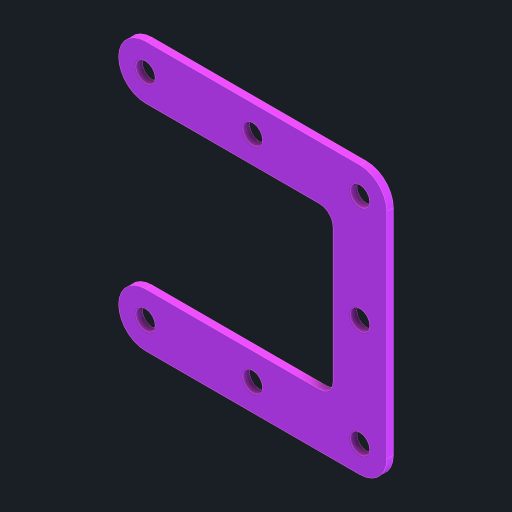
# Autodesk Inventor part: frontgusset
Saved by Autodesk Inventor 2023 (Build 270158000, 158)
## iProperties
Created: 2023-05-11
Part Number: frontgusset
Material: Polycarbonate, Clear
Document SubType Name: Sheet Metal
Designer: reima
Density: 1.2 g/cm^3
Appearance: Magenta
Sheet Metal Rule: Default
Author: reima
Autodesk Inventor part; units mm, degrees
ref_plane "YZ Plane" through (0, 0, 0) normal (1, 0, 0) x (0, 1, 0)
ref_plane "XZ Plane" through (0, 0, 0) normal (0, 1, 0) x (-1, 0, 0)
ref_plane "XY Plane" through (0, 0, 0) normal (0, 0, 1) x (1, 0, 0)
sketch "Sketch1" plane through (0, 0, 0) normal (0, 0, 1) x (1, 0, 0)
  line L0 (-127.5242, -32.3587) -> (-188.9758, -32.3587) projected
  line L1 (-128.9881, -97.1287) -> (-187.5119, -97.1287) projected
  line L2 (-113.8, -97.1287) -> (-113.8, -85.5717) projected
  circle A0 centre (-120.15, -39.9787) radius 2.3114 projected
  circle A1 centre (-120.15, -90.7787) radius 2.3114 projected
  circle A2 centre (-170.95, -90.7787) radius 2.3114 projected
  circle A3 centre (-170.95, -39.9787) radius 2.3114 projected
  circle A4 centre (-158.25, -39.9787) radius 2.3114 projected
  circle A5 centre (-158.25, -90.7787) radius 2.3114 projected
  circle A6 centre (-120.15, -39.9787) radius 6.35
  circle A7 centre (-170.95, -39.9787) radius 6.35
  circle A8 centre (-170.95, -90.7787) radius 6.35
  circle A9 centre (-120.15, -90.7787) radius 6.35
  line L3 (-170.95, -33.6287) -> (-120.15, -33.6287)
  line L4 (-113.8, -39.9787) -> (-113.8, -90.7787)
  line L5 (-120.15, -97.1287) -> (-170.95, -97.1287)
  line L6 (-170.95, -46.3287) -> (-129.675, -46.3287)
  line L7 (-126.5, -49.5037) -> (-126.5, -81.2537)
  line L8 (-129.675, -84.4287) -> (-170.95, -84.4287)
  arc A10 (-126.5, -49.5037) -> (-129.675, -46.3287) centre (-129.675, -49.5037) ccw
  arc A11 (-129.675, -84.4287) -> (-126.5, -81.2537) centre (-129.675, -81.2537) ccw
  circle A12 centre (-170.95, -39.9787) radius 2.3114
  circle A13 centre (-120.15, -39.9787) radius 2.3114
  circle A14 centre (-120.15, -90.7787) radius 2.3114
  circle A15 centre (-170.95, -90.7787) radius 2.3114
  circle A16 centre (-158.25, -90.7787) radius 2.3114
  circle A17 centre (-158.25, -39.9787) radius 2.3114
  point P0 (0, 0)
  dimension "d6" = 12.7
  dimension "d7" = 12.7
  dimension "d8" = 12.7
  dimension "d9" = 12.7
  dimension "d10" = 3.175
  constraints: 12 centre point, 12 end point, 12 point on circle, 10 coincident, 8 tangent, 7 equal radius, 2 point on line, 1 horizontal, 1 perpendicular
  measures "d6" diameter of A6
  measures "d7" diameter of A7
  measures "d8" diameter of A8
  measures "d9" diameter of A9
  measures "d10" radius of A10
extrude "Extrusion1" add sketch "Sketch1" along normal blind 1.5875
sketch "Sketch2" plane through (0, 0, 1.5875) normal (0, 0, 1) x (1, 0, 0)
  circle A0 centre (-158.25, -39.9787) radius 2.3114 projected
  circle A1 centre (-158.25, -39.9787) radius 2.3114
  circle A2 centre (-158.25, -90.7787) radius 2.3114 projected
  circle A3 centre (-158.25, -90.7787) radius 2.3114
  circle A4 centre (-145.55, -90.7787) radius 2.3368
  circle A5 centre (-170.95, -90.7787) radius 2.3114 projected
  circle A6 centre (-145.55, -39.9787) radius 2.3368
  circle A7 centre (-120.15, -65.3787) radius 2.3368
  circle A8 centre (-120.15, -39.9787) radius 2.3114 projected
  line L0 (-113.8, -90.7787) -> (-113.8, -39.9787) projected
  circle A9 centre (-170.95, -39.9787) radius 2.3114 projected
  circle A10 centre (-120.15, -90.7787) radius 2.3114 projected
  point P0 (0, 0)
  dimension "d13" = 4.6736
  dimension "d14" = 25.4
  dimension "d15" = 4.6736
  dimension "d16" = 4.6736
  dimension "d17" = 25.4
  dimension "d18" = 6.35
  dimension "d23" = 25.4
  dimension "d24" = 25.4
  dimension "d25" = 25.4
  constraints: 5 centre point, 2 coincident
  measures "d13" diameter of A4
  measures "d14" distance of A4.centre A5.centre
  measures "d15" diameter of A6
  measures "d16" diameter of A7
  measures "d17" distance of A7.centre A8.centre
  measures "d18" distance from line of L0 A7.centre
  measures "d23" distance of A9.centre A6.centre
  measures "d24" distance of A10.centre A4.centre
  measures "d25" distance of A6.centre A8.centre
extrude "Extrusion2" cut sketch "Sketch2" against normal blind 25.4 contours A4 | A6 | A7
extrude "Extrusion3" add sketch "Sketch2" against normal up to surface (1.5875 mm away) contours A0 | A2
equation "\"BendRadius\" = Thickness"
equation "\"BendReliefWidth\" = Thickness"
equation "\"BendReliefDepth\" = 0.5 * Thickness"
equation "\"CornerReliefSize\" = 4 * Thickness"
equation "\"MinimumRemnant\" = 2 * Thickness"
equation "\"TransitionRadius\" = BendRadius"
equation "\"JacobiRadiusSize\" = BendRadius"
equation "\"GapSize\" = Thickness"
equation "\"Thickness\" = 1.5875"
body "Solid1"
